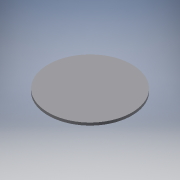
# Autodesk Inventor part: chutecap2
Saved by Autodesk Inventor 2018 (Build 220112000, 112)
## iProperties
Created: 2018-02-05
Part Number: chutecap2
Material: Generic
Document SubType Name: Modeling
Designer: Benedikt
Density: 1 g/cm^3
Appearance: Default
Author: Benedikt
Autodesk Inventor part; units mm, degrees
ref_plane "YZ Plane" through (0, 0, 0) normal (1, 0, 0) x (0, 1, 0)
ref_plane "XZ Plane" through (0, 0, 0) normal (0, 1, 0) x (-1, 0, 0)
ref_plane "XY Plane" through (0, 0, 0) normal (0, 0, 1) x (1, 0, 0)
sketch "Sketch1" plane through (0, 0, 0) normal (0, 0, 1) x (1, 0, 0)
  spline S0 degree 3 poles (-13.5487, 28.6809) (-9.814, 30.4451) (-5.7704, 31.463) (2.4793, 31.8916) (6.6065, 31.2981) (14.4013, 28.5626) (17.9943, 26.4467) (24.1669, 20.9567) (26.6875, 17.6351) (30.3137, 10.2127) (31.3846, 6.1828) (31.9214, -2.0606) (31.3821, -6.1953) (28.7491, -14.0252) (26.6805, -17.6457) (21.272, -23.8898) (17.9838, -26.4538) (10.6096, -30.1771) (6.5941, -31.3007) (-1.6415, -31.9457) (-5.7829, -31.4607) (-13.6468, -28.9307) (-17.294, -26.9098) (-23.6086, -21.5836) (-26.2155, -18.3294) (-30.0353, -11.0047) (-31.2115, -7.0043) (-31.9644, 1.2221) (-31.5339, 5.3696) (-29.1073, 13.266) (-27.1344, 16.9394) (-23.0288, 21.9386) (-21.3492, 23.5762) (-17.6608, 26.4523) (-15.6632, 27.682) (-13.5487, 28.6809) knots -19.990033 -19.990033 -19.990033 -19.990033 -18.750908 -18.750908 -17.511784 -17.511784 -16.272659 -16.272659 -15.033534 -15.033534 -13.79441 -13.79441 -12.555285 -12.555285 -11.316161 -11.316161 -10.077036 -10.077036 -8.837911 -8.837911 -7.598787 -7.598787 -6.359662 -6.359662 -5.120538 -5.120538 -3.881413 -3.881413 -2.642288 -2.642288 -1.403164 -1.403164 -0.701582 -0.701582 0 0 0 0 projected
  point P0 (0, 0)
  point P1 (-13.5487, 28.6809)
  dimension "d0" = 2
extrude "Extrusion1" add sketch "Sketch1" along normal blind 2
body "Solid1"
